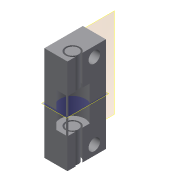
# Autodesk Inventor part: 02_Opentrons_stage_x
Saved by Autodesk Inventor 2019.4 (Build 234330000, 330)
## iProperties
Created: 2020-10-20
Part Number: 02_Opentrons_stage_x
Material: Generic
Document SubType Name: Modeling
Designer: diederichbenedict
Density: 1 g/cm^3
Appearance: Default
Author: diederichbenedict
Autodesk Inventor part; units mm, degrees
ref_plane "YZ Plane" through (0, 0, 0) normal (1, 0, 0) x (0, 1, 0)
ref_plane "XZ Plane" through (0, 0, 0) normal (0, 1, 0) x (-1, 0, 0)
ref_plane "XY Plane" through (0, 0, 0) normal (0, 0, 1) x (1, 0, 0)
ref_plane "Work Plane1" through (-71.5431, 15.4261, 39.8011) normal (1, 0, 0) x (0, -1, 0)
sketch "Sketch1" plane through (-71.5431, 15.4261, 39.8011) normal (1, 0, 0) x (0, -1, 0)
  circle A0 centre (-40.9, -21) radius 3 projected
  circle A1 centre (-1.5, -21) radius 3 projected
  line L0 (-45.9, -13) -> (3.5, -13)
  line L1 (3.5, -13) -> (3.5, -35)
  line L2 (3.5, -35) -> (-45.9, -35)
  line L3 (-45.9, -35) -> (-45.9, -13)
  line L4 (66.8457, -32) -> (-83.1543, -32)
  point P0 (15.4261, 39.8011)
  dimension "d0" = 5
  dimension "d1" = 8
  dimension "d2" = 5
  dimension "d3" = 3
  constraints: 10 end point, 2 horizontal, 2 parallel, 1 perpendicular, 2 other
  measures "d0" distance from line of L3 A0.centre
  measures "d1" distance from line of A0.centre L0
  measures "d2" distance from line of A1.centre L1
  measures "d3" distance between parallel lines of L4 L2
extrude "Extrusion1" add sketch "Sketch1" along normal blind 12
sketch "Sketch2" plane through (-71.5431, 11.9261, 52.8011) normal (0, -1, 0) x (1, 0, 0)
  circle A0 centre (8.688, 16) radius 3 projected
  circle A1 centre (8.688, 16) radius 3.75
  point P0 (71.5431, -52.8011)
  dimension "d6" = 7.5
  constraints: 1 centre point, 1 coincident
  measures "d6" diameter of A1
extrude "Extrusion2" cut sketch "Sketch2" against normal through all contours A0 | A1
ref_plane "Work Plane2" through (-71.5431, 36.6261, 52.8011) normal (0, -1, 0) x (1, 0, 0)
sketch "Sketch3" plane through (-71.5431, 36.6261, 52.8011) normal (0, -1, 0) x (1, 0, 0)
  circle A0 centre (8.688, 16) radius 6 projected
  circle A1 centre (8.688, 16) radius 6.5
  point P0 (71.5431, -52.8011)
  dimension "d9" = 0.5
  constraints: 1 centre point
  measures "d9" radial gap between concentric circles of A0 A1
extrude "Extrusion3" cut sketch "Sketch3" along normal mid plane 20 contours A0 | A1
sketch "Sketch5" plane through (-71.5431, 11.9261, 52.8011) normal (0, 0, -1) x (-1, 0, 0)
  circle A0 centre (-5.5, 42.2) radius 2.1 projected
  arc A1 (-5.5, 5.1) -> (-5.5, 9.3) centre (-5.5, 7.2) ccw projected
  circle A2 centre (-5.5, 42.2) radius 1.45
  circle A3 centre (-5.5, 7.2) radius 1.45
  point P0 (-71.5431, -11.9261)
  dimension "d14" = 2.9
  dimension "d15" = 2.9
  constraints: 2 centre point, 2 coincident
  measures "d14" diameter of A2
  measures "d15" diameter of A3
extrude "Extrusion5" cut sketch "Sketch5" against normal through all contours A2 | A3
body "Solid1"
